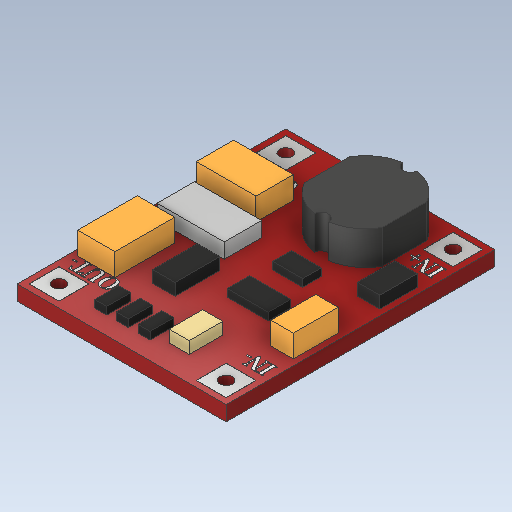
# Autodesk Inventor part: DC-DC RT9266
Saved by Autodesk Inventor 2020.1 (Build 241239000, 239)
## iProperties
Created: 2019-07-20
Part Number: DC-DC RT9266
Material: Generic
Document SubType Name: Modeling
Designer: Petar
Density: 1 g/cm^3
Appearance: Default
Author: Petar
Autodesk Inventor part; units mm, degrees
ref_plane "YZ Plane" through (0, 0, 0) normal (1, 0, 0) x (0, 1, 0)
ref_plane "XZ Plane" through (0, 0, 0) normal (0, 1, 0) x (-1, 0, 0)
ref_plane "XY Plane" through (0, 0, 0) normal (0, 0, 1) x (1, 0, 0)
sketch "Sketch1" plane through (0, 0, 0) normal (0, 1, 0) x (-1, 0, 0)
  line L0 (-7, 9) -> (7, 9)
  line L1 (7, 9) -> (7, -9)
  line L2 (7, -9) -> (-7, -9)
  line L3 (-7, -9) -> (-7, 9)
  line L4 (-7, 9) -> (7, -9) construction
  line L5 (7, 9) -> (-7, -9) construction
  line L6 (13.4742, 17.731) -> (13.4742, -18.9429) construction
  line L7 (13.4742, -18.9429) -> (-16.3947, -18.9429) construction
  line L8 (-16.3947, -18.9429) -> (-16.3947, 17.731) construction
  line L9 (-16.3947, 17.731) -> (13.4742, 17.731) construction
  line L10 (6.6, 8.6) -> (4.6, 8.6)
  line L11 (4.6, 8.6) -> (4.6, 6.6)
  line L12 (4.6, 6.6) -> (6.6, 6.6)
  line L13 (6.6, 6.6) -> (6.6, 8.6)
  line L14 (-4.6, 8.6) -> (-6.6, 8.6)
  line L15 (-6.6, 8.6) -> (-6.6, 6.6)
  line L16 (-6.6, 6.6) -> (-4.6, 6.6)
  line L17 (-4.6, 6.6) -> (-4.6, 8.6)
  line L18 (6.6, -6.6) -> (4.6, -6.6)
  line L19 (4.6, -6.6) -> (4.6, -8.6)
  line L20 (4.6, -8.6) -> (6.6, -8.6)
  line L21 (6.6, -8.6) -> (6.6, -6.6)
  line L22 (-4.6, -6.6) -> (-6.6, -6.6)
  line L23 (-6.6, -6.6) -> (-6.6, -8.6)
  line L24 (-6.6, -8.6) -> (-4.6, -8.6)
  line L25 (-4.6, -8.6) -> (-4.6, -6.6)
  circle A0 centre (5.6, 7.6) radius 0.425
  circle A1 centre (5.6, -7.6) radius 0.425
  line L26 (0, 9) -> (0, -9) construction
  circle A2 centre (-5.6, 7.6) radius 0.425
  circle A3 centre (-5.6, -7.6) radius 0.425
  line L27 (6.6, 5.35) -> (4.1, 5.35)
  line L28 (4.1, 5.35) -> (4.1, 1.35)
  line L29 (4.1, 1.35) -> (6.6, 1.35)
  line L30 (6.6, 1.35) -> (6.6, 5.35)
  line L31 (6.6, -2.6) -> (2.6, -2.6)
  line L32 (2.6, -2.6) -> (2.6, -5.1)
  line L33 (2.6, -5.1) -> (6.6, -5.1)
  line L34 (6.6, -5.1) -> (6.6, -2.6)
  line L35 (0.9981, -4.25) -> (0.9981, -7.25)
  line L36 (-4.1981, -4.25) -> (-4.1981, -7.25)
  arc A4 (-2.0983, -2.7917) -> (-1.1017, -2.7917) centre (-1.6, -2.75) ccw
  arc A5 (-1.1017, -8.7083) -> (-2.0983, -8.7088) centre (-1.6, -8.75) ccw
  arc A6 (0.9981, -4.25) -> (-1.1017, -2.7917) centre (-1.6, -5.75) ccw
  arc A7 (-2.0983, -2.7917) -> (-4.1981, -4.25) centre (-1.6, -5.75) ccw
  arc A8 (-4.1981, -7.25) -> (-2.0983, -8.7083) centre (-1.6, -5.75) ccw
  arc A9 (-1.1017, -8.7083) -> (0.9981, -7.25) centre (-1.6, -5.75) ccw
  line L37 (-1.6, -2.75) -> (-1.6, -8.75) construction
  line L38 (-5.1, 4.1) -> (-6.6, 4.1)
  line L39 (-6.6, 4.1) -> (-6.6, 1.1)
  line L40 (-6.6, 1.1) -> (-5.1, 1.1)
  line L41 (-5.1, 1.1) -> (-5.1, 4.1)
  line L42 (6, 0.625) -> (1.5, 0.625)
  line L43 (1.5, 0.625) -> (1.5, -1.875)
  line L44 (1.5, -1.875) -> (6, -1.875)
  line L45 (6, -1.875) -> (6, 0.625)
  line L46 (6, -0.625) -> (1.5, -0.625) construction
  line L47 (-0.75, -0.375) -> (-2.75, -0.375)
  line L48 (-2.75, -0.375) -> (-2.75, -1.625)
  line L49 (-2.75, -1.625) -> (-0.75, -1.625)
  line L50 (-0.75, -1.625) -> (-0.75, -0.375)
  line L51 (-0.8, 2.725) -> (-3.55, 2.725)
  line L52 (-3.55, 2.725) -> (-3.55, 1.225)
  line L53 (-3.55, 1.225) -> (-0.8, 1.225)
  line L54 (-0.8, 1.225) -> (-0.8, 2.725)
  line L55 (-5.1, -1.7) -> (-6.6, -1.7)
  line L56 (-6.6, -1.7) -> (-6.6, -4.2)
  line L57 (-6.6, -4.2) -> (-5.1, -4.2)
  line L58 (-5.1, -4.2) -> (-5.1, -1.7)
  line L59 (-1.5, 7.325) -> (-2.85, 7.325)
  line L60 (-2.85, 7.325) -> (-2.85, 5.075)
  line L61 (-2.85, 5.075) -> (-1.5, 5.075)
  line L62 (-1.5, 5.075) -> (-1.5, 7.325)
  line L63 (0.1, 7.8) -> (-0.7, 7.8)
  line L64 (-0.7, 7.8) -> (-0.7, 6.2)
  line L65 (-0.7, 6.2) -> (0.1, 6.2)
  line L66 (0.1, 6.2) -> (0.1, 7.8)
  line L67 (0.75, 7.8) -> (1.55, 7.8)
  line L68 (1.55, 7.8) -> (1.55, 6.2)
  line L69 (1.55, 6.2) -> (0.75, 6.2)
  line L70 (0.75, 6.2) -> (0.75, 7.8)
  line L71 (2.2, 7.8) -> (3, 7.8)
  line L72 (3, 7.8) -> (3, 6.2)
  line L73 (3, 6.2) -> (2.2, 6.2)
  line L74 (2.2, 6.2) -> (2.2, 7.8)
  line L75 (2.5, 4.425) -> (1, 4.425)
  line L76 (1, 4.425) -> (1, 1.425)
  line L77 (1, 1.425) -> (2.5, 1.425)
  line L78 (2.5, 1.425) -> (2.5, 4.425)
  point P0 (0, 0)
  dimension "d0" = 14
  dimension "d1" = 18
  dimension "d26" = 2
  dimension "d33" = 0.4
  dimension "d34" = 0.4
  dimension "d35" = 0.4
  dimension "d36" = 0.4
  dimension "d37" = 0.4
  dimension "d38" = 0.4
  dimension "d39" = 0.4
  dimension "d44" = 0.4
  dimension "d45" = 0.85
  dimension "d47" = 1
  dimension "d50" = 1
  dimension "d51" = 1
  dimension "d52" = 1
  dimension "d59" = 2.5
  dimension "d60" = 4
  dimension "d62" = 0.4
  dimension "d63" = 1.25
  dimension "d64" = 4
  dimension "d65" = 2.5
  dimension "d67" = 0.4
  dimension "d68" = 1.5
  dimension "d71" = 0.5
  dimension "d72" = 0.5
  dimension "d76" = 3.25
  dimension "d77" = 3
  dimension "d78" = 3
  dimension "d80" = 3
  dimension "d83" = 1.5
  dimension "d84" = 3
  dimension "d85" = 0.4
  dimension "d86" = 2.5
  dimension "d87" = 4.5
  dimension "d88" = 2.5
  dimension "d89" = 1
  dimension "d90" = 2
  dimension "d91" = 1.25
  dimension "d95" = 2.25
  dimension "d96" = 1
  dimension "d97" = 2.75
  dimension "d98" = 1.5
  dimension "d100" = 1.6
  dimension "d101" = 2.3
  dimension "d102" = 1.5
  dimension "d103" = 2.5
  dimension "d104" = 0.4
  dimension "d105" = 2.8
  dimension "d106" = 1.35
  dimension "d107" = 2.25
  dimension "d110" = 2.35
  dimension "d111" = 1.75
  dimension "d112" = 1.6
  dimension "d113" = 0.8
  dimension "d114" = 0.8
  dimension "d115" = 1.2
  dimension "d117" = 0.65
  dimension "d118" = 0.65
  dimension "d119" = 1.5
  dimension "d120" = 3
  dimension "d122" = 0.8
  dimension "d123" = 1.6
  constraints: 150 end point, 34 parallel, 19 horizontal, 17 perpendicular, 15 point on circle, 10 centre point, 10 equal length, 7 midpoint, 5 vertical, 4 collinear, 4 equal radius, 2 symmetric about line, 5 other
  measures "d0" distance of L1.end L2.end
  measures "d1" distance of L0.end L1.end
  measures "d26" distance of L11.end L10.end
  measures "d33" distance between parallel lines of L0 L10
  measures "d34" distance between parallel lines of L0 L14
  measures "d35" distance between parallel lines of L3 L15
  measures "d36" distance between parallel lines of L1 L13
  measures "d37" distance between parallel lines of L1 L21
  measures "d38" distance between parallel lines of L2 L20
  measures "d39" distance between parallel lines of L2 L24
  measures "d44" distance between parallel lines of L3 L23
  measures "d45" diameter of A0
  measures "d47" distance from line of L13 A0.centre
  measures "d50" distance from line of L10 A0.centre
  measures "d51" distance from line of L21 A1.centre
  measures "d52" distance from line of L20 A1.centre
  measures "d59" distance of L29.end L28.end
  measures "d60" distance of L28.end L27.end
  measures "d62" distance between parallel lines of L1 L30
  measures "d63" distance between parallel lines of L12 L27
  measures "d64" distance of L33.end L32.end
  measures "d65" distance of L32.end L31.end
  measures "d67" distance between parallel lines of L1 L34
  measures "d68" distance between parallel lines of L18 L33
  measures "d71" radius of A4
  measures "d72" radius of A5
  measures "d76" distance from line of L2 A6.centre
  measures "d77" distance from line of L25 A6.centre
  measures "d78" distance of L35.start L35.end
  measures "d80" radius of A6
  measures "d83" distance of L40.end L39.end
  measures "d84" distance of L39.end L38.end
  measures "d85" distance between parallel lines of L3 L39
  measures "d86" distance between parallel lines of L16 L38
  measures "d87" distance of L44.end L43.end
  measures "d88" distance of L43.end L42.end
  measures "d89" distance between parallel lines of L1 L45
  measures "d90" distance of L49.end L48.end
  measures "d91" distance of L48.end L47.end
  measures "d95" distance between parallel lines of L43 L50
  measures "d96" distance between parallel lines of L42 L47
  measures "d97" distance of L53.end L52.end
  measures "d98" distance of L52.end L51.end
  measures "d100" distance between parallel lines of L47 L53
  measures "d101" distance between parallel lines of L43 L54
  measures "d102" distance of L57.end L56.end
  measures "d103" distance of L56.end L55.end
  measures "d104" distance between parallel lines of L3 L56
  measures "d105" distance between parallel lines of L40 L55
  measures "d106" distance of L61.end L60.end
  measures "d107" distance of L60.end L59.end
  measures "d110" distance between parallel lines of L51 L61
  measures "d111" distance between parallel lines of L17 L60
  measures "d112" distance of L64.end L63.end
  measures "d113" distance of L64.end L65.end
  measures "d114" distance between parallel lines of L62 L64
  measures "d115" distance between parallel lines of L0 L63
  measures "d117" distance between parallel lines of L66 L70
  measures "d118" distance between parallel lines of L68 L74
  measures "d119" distance of L77.end L76.end
  measures "d120" distance of L76.end L75.end
  measures "d122" distance between parallel lines of L42 L77
  measures "d123" distance between parallel lines of L28 L78
extrude "Extrusion1" add sketch "Sketch1" against normal blind 1 contours L0 L1 L2 L3 | L13 L12 L11 L10 | L17 L16 L15 L14 | L21 L20 L19 L18 | L25 L24 L23 L22 | L30 L29 L28 L27 | L34 L33 L32 L31 | L35 A9 A5 A8 L36 A7 A4 A6 | L41 L40 L39 L38 | L45 L44 L43 L42 | L50 L49 L48 L47 | L54 L53 L52 L51 | L58 L57 L56 L55 | L62 L61 L60 L59 | L66 L65 L64 L63 | L67 L68 L69 L70 | L71 L72 L73 L74 | L78 L77 L76 L75
extrude "Extrusion2" add sketch "Sketch1" along normal blind 0.01 contours L13 L12 L11 L10 | L17 L16 L15 L14 | L21 L20 L19 L18 | L25 L24 L23 L22
extrude "Extrusion3" add sketch "Sketch1" along normal blind 1.5 contours L30 L29 L28 L27 | L34 L33 L32 L31 | L41 L40 L39 L38
extrude "Extrusion4" add sketch "Sketch1" along normal blind 1 contours L45 L44 L43 L42
extrude "Extrusion5" add sketch "Sketch1" along normal blind 0.8 contours L58 L57 L56 L55 | L62 L61 L60 L59 | L78 L77 L76 L75
extrude "Extrusion6" add sketch "Sketch1" along normal blind 0.5 contours L50 L49 L48 L47 | L54 L53 L52 L51 | L66 L65 L64 L63 | L67 L68 L69 L70 | L71 L72 L73 L74
extrude "Extrusion7" add sketch "Sketch1" along normal blind 2.25 contours L35 A9 A5 A8 L36 A7 A4 A6
sketch "Sketch2" plane through (0, 0, 0) normal (0, 1, 0) x (1, 0, 0)
  line L0 (6.6, -6.1) -> (4.6, -6.1) construction
  line L1 (4.6, -6.1) -> (4.6, -5) construction
  line L2 (4.6, -5) -> (6.6, -5) construction
  line L3 (6.6, -5) -> (6.6, -6.1) construction
  line L4 (6.6, -8.6) -> (6.6, -6.6) construction
  line L5 (6.6, -6.6) -> (4.6, -6.6) construction
  line L6 (6.6, 5.217) -> (4.6, 5.217) construction
  line L7 (4.6, 5.217) -> (4.6, 6.1) construction
  line L8 (4.6, 6.1) -> (6.6, 6.1) construction
  line L9 (6.6, 6.1) -> (6.6, 5.217) construction
  line L10 (6.6, 6.6) -> (6.6, 8.6) construction
  line L11 (4.6, 6.6) -> (6.6, 6.6) construction
  line L12 (-3.0572, 6.1) -> (-3.0572, 5.217) construction
  line L13 (-3.0572, 5.217) -> (-6.6, 5.217) construction
  line L14 (-6.6, 5.217) -> (-6.6, 6.1) construction
  line L15 (-6.6, 6.1) -> (-3.0572, 6.1) construction
  line L16 (-6.6, 8.6) -> (-6.6, 6.6) construction
  line L17 (-3.0572, -5.7507) -> (-3.0572, -6.4) construction
  line L18 (-3.0572, -6.4) -> (-6.6, -6.4) construction
  line L19 (-6.6, -6.4) -> (-6.6, -5.7507) construction
  line L20 (-6.6, -5.7507) -> (-3.0572, -5.7507) construction
  line L21 (-4.6, -6.6) -> (-6.6, -6.6) construction
  line L22 (6.5616, -5.108) -> (6.129, -5.108)
  line L23 (6.129, -5.108) -> (6.129, -5.1714)
  spline S0 degree 2 poles (6.129, -5.1714) (6.1798, -5.1705) (6.228, -5.1874) (6.2423, -5.2365) (6.2414, -5.2847) knots 0 0 0 1 2 3 3 3
  line L24 (6.2414, -5.2847) -> (6.2414, -5.9216)
  spline S1 degree 2 poles (6.2414, -5.9216) (6.2423, -5.9707) (6.228, -6.0197) (6.1798, -6.0358) (6.129, -6.0349) knots 0 0 0 1 2 3 3 3
  line L25 (6.129, -6.0349) -> (6.129, -6.0991)
  line L26 (6.129, -6.0991) -> (6.5616, -6.0991)
  line L27 (6.5616, -6.0991) -> (6.5616, -6.0349)
  spline S2 degree 2 poles (6.5616, -6.0349) (6.5108, -6.0358) (6.4626, -6.0197) (6.4483, -5.9707) (6.4492, -5.9216) knots 0 0 0 1 2 3 3 3
  line L28 (6.4492, -5.9216) -> (6.4492, -5.2847)
  spline S3 degree 2 poles (6.4492, -5.2847) (6.4483, -5.2365) (6.4626, -5.1874) (6.5108, -5.1705) (6.5616, -5.1714) knots 0 0 0 1 2 3 3 3
  line L29 (6.5616, -5.1714) -> (6.5616, -5.108)
  line L30 (6.0541, -6.0991) -> (6.0541, -6.0349)
  spline S4 degree 2 poles (6.0541, -6.0349) (6.0086, -6.0358) (5.9649, -6.0215) (5.9515, -5.9733) (5.9524, -5.9243) knots 0 0 0 1 2 3 3 3
  line L31 (5.9524, -5.9243) -> (5.9524, -5.2847)
  spline S5 degree 2 poles (5.9524, -5.2847) (5.9506, -5.2133) (5.9872, -5.1696) (6.0523, -5.1714) knots 0 0 0 1 2 2 2
  line L32 (6.0523, -5.1714) -> (6.0523, -5.108)
  line L33 (6.0523, -5.108) -> (5.7641, -5.108)
  line L34 (5.7641, -5.108) -> (5.7641, -5.1714)
  spline S6 degree 2 poles (5.7641, -5.1714) (5.8293, -5.1696) (5.8658, -5.2133) (5.864, -5.2847) knots 0 0 0 1 2 2 2
  line L35 (5.864, -5.2847) -> (5.864, -5.9046)
  line L36 (5.864, -5.9046) -> (5.8614, -5.9046)
  line L37 (5.8614, -5.9046) -> (5.4207, -5.0938)
  line L38 (5.4207, -5.0938) -> (5.2806, -5.0938)
  line L39 (5.2806, -5.0938) -> (5.2806, -5.9216)
  spline S7 degree 2 poles (5.2806, -5.9216) (5.2824, -5.9938) (5.2441, -6.0376) (5.1834, -6.0349) knots 0 0 0 1 2 2 2
  line L40 (5.1834, -6.0349) -> (5.1834, -6.0991)
  line L41 (5.1834, -6.0991) -> (5.4724, -6.0991)
  line L42 (5.4724, -6.0991) -> (5.4724, -6.0349)
  spline S8 degree 2 poles (5.4724, -6.0349) (5.4064, -6.0376) (5.3663, -5.9938) (5.3681, -5.9216) knots 0 0 0 1 2 2 2
  line L43 (5.3681, -5.9216) -> (5.3681, -5.3694)
  line L44 (5.3681, -5.3694) -> (5.3707, -5.3694)
  line L45 (5.3707, -5.3694) -> (5.7624, -6.0991)
  line L46 (5.7624, -6.0991) -> (6.0541, -6.0991)
  line L47 (5.1004, -5.3944) -> (4.8239, -5.3944)
  line L48 (4.8239, -5.3944) -> (4.8239, -5.4827)
  line L49 (4.8239, -5.4827) -> (5.1004, -5.4827)
  line L50 (5.1004, -5.4827) -> (5.1004, -5.3944)
  line L51 (6.5616, 6.209) -> (6.129, 6.209)
  line L52 (6.129, 6.209) -> (6.129, 6.1456)
  spline S9 degree 2 poles (6.129, 6.1456) (6.1798, 6.1465) (6.228, 6.1296) (6.2423, 6.0805) (6.2414, 6.0323) knots 0 0 0 1 2 3 3 3
  line L53 (6.2414, 6.0323) -> (6.2414, 5.3954)
  spline S10 degree 2 poles (6.2414, 5.3954) (6.2423, 5.3464) (6.228, 5.2973) (6.1798, 5.2812) (6.129, 5.2821) knots 0 0 0 1 2 3 3 3
  line L54 (6.129, 5.2821) -> (6.129, 5.2179)
  line L55 (6.129, 5.2179) -> (6.5616, 5.2179)
  line L56 (6.5616, 5.2179) -> (6.5616, 5.2821)
  spline S11 degree 2 poles (6.5616, 5.2821) (6.5108, 5.2812) (6.4626, 5.2973) (6.4483, 5.3464) (6.4492, 5.3954) knots 0 0 0 1 2 3 3 3
  line L57 (6.4492, 5.3954) -> (6.4492, 6.0323)
  spline S12 degree 2 poles (6.4492, 6.0323) (6.4483, 6.0805) (6.4626, 6.1296) (6.5108, 6.1465) (6.5616, 6.1456) knots 0 0 0 1 2 3 3 3
  line L58 (6.5616, 6.1456) -> (6.5616, 6.209)
  line L59 (6.0541, 5.2179) -> (6.0541, 5.2821)
  spline S13 degree 2 poles (6.0541, 5.2821) (6.0086, 5.2812) (5.9649, 5.2955) (5.9515, 5.3437) (5.9524, 5.3927) knots 0 0 0 1 2 3 3 3
  line L60 (5.9524, 5.3927) -> (5.9524, 6.0323)
  spline S14 degree 2 poles (5.9524, 6.0323) (5.9506, 6.1037) (5.9872, 6.1474) (6.0523, 6.1456) knots 0 0 0 1 2 2 2
  line L61 (6.0523, 6.1456) -> (6.0523, 6.209)
  line L62 (6.0523, 6.209) -> (5.7641, 6.209)
  line L63 (5.7641, 6.209) -> (5.7641, 6.1456)
  spline S15 degree 2 poles (5.7641, 6.1456) (5.8293, 6.1474) (5.8658, 6.1037) (5.864, 6.0323) knots 0 0 0 1 2 2 2
  line L64 (5.864, 6.0323) -> (5.864, 5.4124)
  line L65 (5.864, 5.4124) -> (5.8614, 5.4124)
  line L66 (5.8614, 5.4124) -> (5.4207, 6.2233)
  line L67 (5.4207, 6.2233) -> (5.2806, 6.2233)
  line L68 (5.2806, 6.2233) -> (5.2806, 5.3954)
  spline S16 degree 2 poles (5.2806, 5.3954) (5.2824, 5.3232) (5.2441, 5.2795) (5.1834, 5.2821) knots 0 0 0 1 2 2 2
  line L69 (5.1834, 5.2821) -> (5.1834, 5.2179)
  line L70 (5.1834, 5.2179) -> (5.4724, 5.2179)
  line L71 (5.4724, 5.2179) -> (5.4724, 5.2821)
  spline S17 degree 2 poles (5.4724, 5.2821) (5.4064, 5.2795) (5.3663, 5.3232) (5.3681, 5.3954) knots 0 0 0 1 2 2 2
  line L72 (5.3681, 5.3954) -> (5.3681, 5.9476)
  line L73 (5.3681, 5.9476) -> (5.3707, 5.9476)
  line L74 (5.3707, 5.9476) -> (5.7624, 5.2179)
  line L75 (5.7624, 5.2179) -> (6.0541, 5.2179)
  line L76 (4.8525, 5.5524) -> (4.8525, 5.8093)
  line L77 (4.8525, 5.8093) -> (5.1004, 5.8093)
  line L78 (5.1004, 5.8093) -> (5.1004, 5.9012)
  line L79 (5.1004, 5.9012) -> (4.8525, 5.9012)
  line L80 (4.8525, 5.9012) -> (4.8525, 6.1742)
  line L81 (4.8525, 6.1742) -> (4.7588, 6.1742)
  line L82 (4.7588, 6.1742) -> (4.7588, 5.9012)
  line L83 (4.7588, 5.9012) -> (4.5108, 5.9012)
  line L84 (4.5108, 5.9012) -> (4.5108, 5.8093)
  line L85 (4.5108, 5.8093) -> (4.7588, 5.8093)
  line L86 (4.7588, 5.8093) -> (4.7588, 5.5524)
  line L87 (4.7588, 5.5524) -> (4.8525, 5.5524)
  spline S18 degree 2 poles (-3.6758, 6.2464) (-3.774, 6.2464) (-3.9301, 6.1911) (-3.9863, 6.1296) knots 0 0 0 1 2 2 2
  spline S19 degree 2 poles (-3.9863, 6.1296) (-4.0416, 6.0707) (-4.1058, 5.8753) (-4.1067, 5.7308) knots 0 0 0 1 2 2 2
  spline S20 degree 2 poles (-4.1067, 5.7308) (-4.1076, 5.6577) (-4.0773, 5.4819) (-3.9889, 5.3223) (-3.8168, 5.2188) (-3.6758, 5.217) knots 0 0 0 1 2 3 4 4 4
  spline S21 degree 2 poles (-3.6758, 5.217) (-3.5447, 5.2179) (-3.377, 5.3098) (-3.2833, 5.4614) (-3.2459, 5.6416) (-3.2467, 5.7308) knots 0 0 0 1 2 3 4 4 4
  spline S22 degree 2 poles (-3.2467, 5.7308) (-3.2476, 5.8753) (-3.3119, 6.0707) (-3.3672, 6.1296) knots 0 0 0 1 2 2 2
  spline S23 degree 2 poles (-3.3672, 6.1296) (-3.4323, 6.1992) (-3.5938, 6.2482) (-3.6758, 6.2464) knots 0 0 0 1 2 2 2
  spline S24 degree 2 poles (-3.6758, 5.2857) (-3.7463, 5.2866) (-3.8319, 5.366) (-3.8748, 5.4962) (-3.8899, 5.6523) (-3.889, 5.7308) knots 0 0 0 1 2 3 4 4 4
  spline S25 degree 2 poles (-3.889, 5.7308) (-3.8899, 5.8049) (-3.8748, 5.9592) (-3.831, 6.093) (-3.7445, 6.176) (-3.674, 6.1769) knots 0 0 0 1 2 3 4 4 4
  spline S26 degree 2 poles (-3.674, 6.1769) (-3.6054, 6.176) (-3.5206, 6.0939) (-3.4769, 5.961) (-3.4608, 5.8058) (-3.4617, 5.7308) knots 0 0 0 1 2 3 4 4 4
  spline S27 degree 2 poles (-3.4617, 5.7308) (-3.4608, 5.6523) (-3.476, 5.4953) (-3.5197, 5.3651) (-3.6054, 5.2866) (-3.6758, 5.2857) knots 0 0 0 1 2 3 4 4 4
  spline S28 degree 2 poles (-4.509, 5.4133) (-4.5081, 5.3624) (-4.5197, 5.3133) (-4.5581, 5.2991) (-4.5991, 5.3) knots 0 0 0 1 2 3 3 3
  line L88 (-4.5991, 5.3) -> (-4.5991, 5.2357)
  line L89 (-4.5991, 5.2357) -> (-4.203, 5.2357)
  line L90 (-4.203, 5.2357) -> (-4.203, 5.3)
  spline S29 degree 2 poles (-4.203, 5.3) (-4.2664, 5.2973) (-4.3012, 5.341) (-4.2994, 5.4133) knots 0 0 0 1 2 2 2
  line L91 (-4.2994, 5.4133) -> (-4.2994, 5.8932)
  spline S30 degree 2 poles (-4.2994, 5.8932) (-4.2976, 5.9967) (-4.3475, 6.1555) (-4.5001, 6.2456) (-4.6526, 6.2464) knots 0 0 0 1 2 3 3 3
  spline S31 degree 2 poles (-4.6526, 6.2464) (-4.7606, 6.2456) (-4.8881, 6.176) (-4.9488, 6.068) (-4.9675, 5.9503) (-4.9666, 5.9012) knots 0 0 0 1 2 3 4 4 4
  line L92 (-4.9666, 5.9012) -> (-4.9666, 5.4133)
  spline S32 degree 2 poles (-4.9666, 5.4133) (-4.9649, 5.341) (-4.9988, 5.2973) (-5.0558, 5.3) knots 0 0 0 1 2 2 2
  line L93 (-5.0558, 5.3) -> (-5.0558, 5.2357)
  line L94 (-5.0558, 5.2357) -> (-4.7882, 5.2357)
  line L95 (-4.7882, 5.2357) -> (-4.7882, 5.3)
  spline S33 degree 2 poles (-4.7882, 5.3) (-4.8275, 5.2991) (-4.8658, 5.3142) (-4.8792, 5.3633) (-4.8783, 5.4133) knots 0 0 0 1 2 3 3 3
  line L96 (-4.8783, 5.4133) -> (-4.8783, 5.8905)
  spline S34 degree 2 poles (-4.8783, 5.8905) (-4.8792, 5.9235) (-4.8703, 6.0118) (-4.8355, 6.0975) (-4.7588, 6.1546) (-4.6928, 6.1555) knots 0 0 0 1 2 3 4 4 4
  spline S35 degree 2 poles (-4.6928, 6.1555) (-4.608, 6.1537) (-4.5295, 6.0654) (-4.5072, 5.9423) (-4.509, 5.8878) knots 0 0 0 1 2 3 3 3
  line L97 (-4.509, 5.8878) -> (-4.509, 5.4133)
  spline S36 degree 2 poles (-5.7062, 5.3151) (-5.7463, 5.3133) (-5.79, 5.3321) (-5.8168, 5.4061) (-5.8302, 5.4873) knots 0 0 0 1 2 3 3 3
  line L98 (-5.8302, 5.4873) -> (-5.9095, 5.4873)
  line L99 (-5.9095, 5.4873) -> (-5.8774, 5.2357)
  line L100 (-5.8774, 5.2357) -> (-5.1335, 5.2357)
  line L101 (-5.1335, 5.2357) -> (-5.1004, 5.4873)
  line L102 (-5.1004, 5.4873) -> (-5.1807, 5.4873)
  spline S37 degree 2 poles (-5.1807, 5.4873) (-5.1941, 5.4061) (-5.2209, 5.333) (-5.2637, 5.3133) (-5.3029, 5.3151) knots 0 0 0 1 2 3 3 3
  line L103 (-5.3029, 5.3151) -> (-5.402, 5.3151)
  line L104 (-5.402, 5.3151) -> (-5.402, 6.0502)
  spline S38 degree 2 poles (-5.402, 6.0502) (-5.4029, 6.0993) (-5.3886, 6.1483) (-5.3368, 6.1644) (-5.2824, 6.1635) knots 0 0 0 1 2 3 3 3
  line L105 (-5.2824, 6.1635) -> (-5.2824, 6.2268)
  line L106 (-5.2824, 6.2268) -> (-5.7285, 6.2268)
  line L107 (-5.7285, 6.2268) -> (-5.7285, 6.1635)
  spline S39 degree 2 poles (-5.7285, 6.1635) (-5.674, 6.1644) (-5.6223, 6.1483) (-5.608, 6.0993) (-5.6089, 6.0502) knots 0 0 0 1 2 3 3 3
  line L108 (-5.6089, 6.0502) -> (-5.6089, 5.3151)
  line L109 (-5.6089, 5.3151) -> (-5.7062, 5.3151)
  line L110 (-6.2164, 5.5703) -> (-6.2164, 5.8272)
  line L111 (-6.2164, 5.8272) -> (-5.9684, 5.8272)
  line L112 (-5.9684, 5.8272) -> (-5.9684, 5.9191)
  line L113 (-5.9684, 5.9191) -> (-6.2164, 5.9191)
  line L114 (-6.2164, 5.9191) -> (-6.2164, 6.192)
  line L115 (-6.2164, 6.192) -> (-6.3101, 6.192)
  line L116 (-6.3101, 6.192) -> (-6.3101, 5.9191)
  line L117 (-6.3101, 5.9191) -> (-6.5581, 5.9191)
  line L118 (-6.5581, 5.9191) -> (-6.5581, 5.8272)
  line L119 (-6.5581, 5.8272) -> (-6.3101, 5.8272)
  line L120 (-6.3101, 5.8272) -> (-6.3101, 5.5703)
  line L121 (-6.3101, 5.5703) -> (-6.2164, 5.5703)
  spline S40 degree 2 poles (-3.988, -5.3706) (-4.0862, -5.3706) (-4.2423, -5.4259) (-4.2985, -5.4874) knots 0 0 0 1 2 2 2
  spline S41 degree 2 poles (-4.2985, -5.4874) (-4.3538, -5.5463) (-4.418, -5.7417) (-4.4189, -5.8862) knots 0 0 0 1 2 2 2
  spline S42 degree 2 poles (-4.4189, -5.8862) (-4.4198, -5.9593) (-4.3895, -6.1351) (-4.3012, -6.2947) (-4.129, -6.3982) (-3.988, -6.4) knots 0 0 0 1 2 3 4 4 4
  spline S43 degree 2 poles (-3.988, -6.4) (-3.8569, -6.3991) (-3.6892, -6.3072) (-3.5955, -6.1556) (-3.5581, -5.9754) (-3.559, -5.8862) knots 0 0 0 1 2 3 4 4 4
  spline S44 degree 2 poles (-3.559, -5.8862) (-3.5599, -5.7417) (-3.6241, -5.5463) (-3.6794, -5.4874) knots 0 0 0 1 2 2 2
  spline S45 degree 2 poles (-3.6794, -5.4874) (-3.7445, -5.4178) (-3.906, -5.3688) (-3.988, -5.3706) knots 0 0 0 1 2 2 2
  spline S46 degree 2 poles (-3.988, -6.3313) (-4.0585, -6.3304) (-4.1442, -6.251) (-4.187, -6.1208) (-4.2021, -5.9647) (-4.2012, -5.8862) knots 0 0 0 1 2 3 4 4 4
  spline S47 degree 2 poles (-4.2012, -5.8862) (-4.2021, -5.8121) (-4.187, -5.6578) (-4.1433, -5.524) (-4.0567, -5.441) (-3.9863, -5.4401) knots 0 0 0 1 2 3 4 4 4
  spline S48 degree 2 poles (-3.9863, -5.4401) (-3.9176, -5.441) (-3.8328, -5.5231) (-3.7891, -5.656) (-3.7731, -5.8112) (-3.774, -5.8862) knots 0 0 0 1 2 3 4 4 4
  spline S49 degree 2 poles (-3.774, -5.8862) (-3.7731, -5.9647) (-3.7882, -6.1217) (-3.8319, -6.2519) (-3.9176, -6.3304) (-3.988, -6.3313) knots 0 0 0 1 2 3 4 4 4
  spline S50 degree 2 poles (-4.8212, -6.2037) (-4.8203, -6.2546) (-4.8319, -6.3037) (-4.8703, -6.3179) (-4.9113, -6.317) knots 0 0 0 1 2 3 3 3
  line L122 (-4.9113, -6.317) -> (-4.9113, -6.3813)
  line L123 (-4.9113, -6.3813) -> (-4.5153, -6.3813)
  line L124 (-4.5153, -6.3813) -> (-4.5153, -6.317)
  spline S51 degree 2 poles (-4.5153, -6.317) (-4.5786, -6.3197) (-4.6134, -6.276) (-4.6116, -6.2037) knots 0 0 0 1 2 2 2
  line L125 (-4.6116, -6.2037) -> (-4.6116, -5.7238)
  spline S52 degree 2 poles (-4.6116, -5.7238) (-4.6098, -5.6203) (-4.6598, -5.4616) (-4.8123, -5.3715) (-4.9649, -5.3706) knots 0 0 0 1 2 3 3 3
  spline S53 degree 2 poles (-4.9649, -5.3706) (-5.0728, -5.3715) (-5.2004, -5.441) (-5.261, -5.549) (-5.2798, -5.6667) (-5.2789, -5.7158) knots 0 0 0 1 2 3 4 4 4
  line L126 (-5.2789, -5.7158) -> (-5.2789, -6.2037)
  spline S54 degree 2 poles (-5.2789, -6.2037) (-5.2771, -6.276) (-5.311, -6.3197) (-5.3681, -6.317) knots 0 0 0 1 2 2 2
  line L127 (-5.3681, -6.317) -> (-5.3681, -6.3813)
  line L128 (-5.3681, -6.3813) -> (-5.1004, -6.3813)
  line L129 (-5.1004, -6.3813) -> (-5.1004, -6.317)
  spline S55 degree 2 poles (-5.1004, -6.317) (-5.1397, -6.3179) (-5.1781, -6.3028) (-5.1914, -6.2537) (-5.1905, -6.2037) knots 0 0 0 1 2 3 3 3
  line L130 (-5.1905, -6.2037) -> (-5.1905, -5.7265)
  spline S56 degree 2 poles (-5.1905, -5.7265) (-5.1914, -5.6935) (-5.1825, -5.6052) (-5.1477, -5.5195) (-5.071, -5.4624) (-5.005, -5.4616) knots 0 0 0 1 2 3 4 4 4
  spline S57 degree 2 poles (-5.005, -5.4616) (-4.9202, -5.4633) (-4.8417, -5.5517) (-4.8194, -5.6748) (-4.8212, -5.7292) knots 0 0 0 1 2 3 3 3
  line L131 (-4.8212, -5.7292) -> (-4.8212, -6.2037)
  spline S58 degree 2 poles (-6.0184, -6.3019) (-6.0585, -6.3037) (-6.1022, -6.2849) (-6.129, -6.2109) (-6.1424, -6.1297) knots 0 0 0 1 2 3 3 3
  line L132 (-6.1424, -6.1297) -> (-6.2218, -6.1297)
  line L133 (-6.2218, -6.1297) -> (-6.1897, -6.3813)
  line L134 (-6.1897, -6.3813) -> (-5.4457, -6.3813)
  line L135 (-5.4457, -6.3813) -> (-5.4127, -6.1297)
  line L136 (-5.4127, -6.1297) -> (-5.493, -6.1297)
  spline S59 degree 2 poles (-5.493, -6.1297) (-5.5063, -6.2109) (-5.5331, -6.284) (-5.5759, -6.3037) (-5.6152, -6.3019) knots 0 0 0 1 2 3 3 3
  line L137 (-5.6152, -6.3019) -> (-5.7142, -6.3019)
  line L138 (-5.7142, -6.3019) -> (-5.7142, -5.5668)
  spline S60 degree 2 poles (-5.7142, -5.5668) (-5.7151, -5.5178) (-5.7008, -5.4687) (-5.6491, -5.4526) (-5.5946, -5.4535) knots 0 0 0 1 2 3 3 3
  line L139 (-5.5946, -5.4535) -> (-5.5946, -5.3902)
  line L140 (-5.5946, -5.3902) -> (-6.0407, -5.3902)
  line L141 (-6.0407, -5.3902) -> (-6.0407, -5.4535)
  spline S61 degree 2 poles (-6.0407, -5.4535) (-5.9863, -5.4526) (-5.9345, -5.4687) (-5.9202, -5.5178) (-5.9211, -5.5668) knots 0 0 0 1 2 3 3 3
  line L142 (-5.9211, -5.5668) -> (-5.9211, -6.3019)
  line L143 (-5.9211, -6.3019) -> (-6.0184, -6.3019)
  line L144 (-6.2806, -5.6765) -> (-6.5572, -5.6765)
  line L145 (-6.5572, -5.6765) -> (-6.5572, -5.7649)
  line L146 (-6.5572, -5.7649) -> (-6.2806, -5.7649)
  line L147 (-6.2806, -5.7649) -> (-6.2806, -5.6765)
  point P0 (0, 0)
  dimension "d138" = 0.5
  dimension "d139" = 0.5
  dimension "d140" = 0.2
  constraints: 6 collinear, 8 other
  measures "d138" distance between parallel lines of L0 L5
  measures "d139" distance between parallel lines of L11 L8
  measures "d140" distance between parallel lines of L18 L21
emboss "Emboss1" sketch "Sketch2" operation add depth 0.01 direction (0, -1, 0)
equation "\"d34\" = d33"
equation "\"d35\" = d33"
equation "\"d36\" = d33"
equation "\"d37\" = d33"
equation "\"d38\" = d33"
equation "\"d39\" = d33"
equation "\"d44\" = d33"
equation "\"d50\" = d47"
equation "\"d51\" = d47"
equation "\"d52\" = d47"
equation "\"d85\" = d35"
equation "\"d104\" = d85"
body "Solid1"
